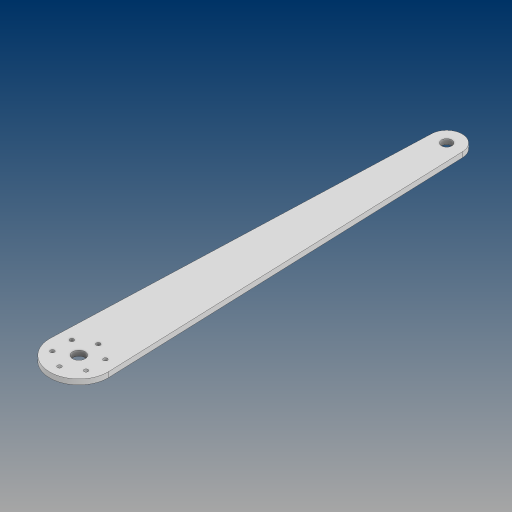
# Autodesk Inventor part: DragBarLinkage3 Bar1
Saved by Autodesk Inventor 2024.3 (Build 283343000, 343)
## iProperties
Created: 2024-07-08
Part Number: DragBarLinkage3 Bar1
Material: Generic
Document SubType Name: Modeling
Designer: Kenji
Density: 1 g/cm^3
Appearance: Default
Author: Kenji
Autodesk Inventor part; units mm, degrees
ref_plane "YZ Plane" through (0, 0, 0) normal (1, 0, 0) x (0, 1, 0)
ref_plane "XZ Plane" through (0, 0, 0) normal (0, 1, 0) x (-1, 0, 0)
ref_plane "XY Plane" through (0, 0, 0) normal (0, 0, 1) x (1, 0, 0)
sketch "Sketch1" plane through (0, 0, 0) normal (0, 1, 0) x (-1, 0, 0)
  line L0 (0, 0) -> (0, -452.12) construction
  circle A0 centre (0, -452.12) radius 6.35
  circle A1 centre (0, 0) radius 7.62
  circle A2 centre (0, 0) radius 29.337 construction
  circle A3 centre (0, 0) radius 35.687 construction
  circle A4 centre (0, -452.12) radius 19.05 construction
  circle A5 centre (0, 0) radius 23.8125 construction
  circle A6 centre (0, -23.8125) radius 2.413
  circle A7 centre (20.6222, -11.9063) radius 2.413
  circle A8 centre (20.6222, 11.9062) radius 2.413
  circle A9 centre (0, 23.8125) radius 2.413
  circle A10 centre (-20.6222, 11.9063) radius 2.413
  circle A11 centre (-20.6222, -11.9062) radius 2.413
  line L1 (35.6628, -1.3132) -> (19.0371, -452.821)
  line L2 (-35.6628, -1.3132) -> (-19.0371, -452.821)
  arc A12 (35.6628, -1.3132) -> (-35.6628, -1.3132) centre (0, 0) ccw
  arc A13 (-19.0371, -452.821) -> (19.0371, -452.821) centre (0, -452.12) ccw
  dimension "d6" = 47.625
  dimension "d0" = 452.12
  dimension "d1" = 12.7
  dimension "d2" = 15.24
  dimension "d3" = 58.674
  dimension "d4" = 6.35
  dimension "d5" = 12.7
  dimension "d7" = 4.826
  dimension "d10" = 360
  constraints: 13 centre point, 8 point on circle, 6 end point, 6 tangent, 5 coincident, 2 vertical alignment, 1 vertical, 15 other
  measures "d0" distance of L0.start L0.end
  measures "d1" diameter of A0
  measures "d2" diameter of A1
  measures "d3" diameter of A2
  measures "d4" radial gap between concentric circles of A2 A3
  measures "d5" radial gap between concentric circles of A0 A4
  measures "d7" diameter of A6
extrude "Extrusion1" add sketch "Sketch1" along normal blind 6.35
body "Solid1"
